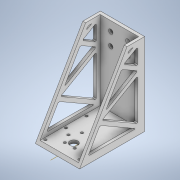
# Autodesk Inventor part: Top
Saved by Autodesk Inventor 2020 (Build 240168000, 168)
## iProperties
Created: 2019-08-01
Part Number: Top
Material: Generic
Document SubType Name: Modeling
Designer: Alex
Density: 1 g/cm^3
Appearance: Default
Author: Alex
Autodesk Inventor part; units mm, degrees
ref_plane "YZ Plane" through (0, 0, 0) normal (1, 0, 0) x (0, 1, 0)
ref_plane "XZ Plane" through (0, 0, 0) normal (0, 1, 0) x (-1, 0, 0)
ref_plane "XY Plane" through (0, 0, 0) normal (0, 0, 1) x (1, 0, 0)
sketch "Sketch1" plane through (0, 0, 0) normal (0, 1, 0) x (-1, 0, 0)
  line L0 (-35, -50) -> (35, -50)
  line L1 (35, -50) -> (35, 50)
  line L2 (35, 50) -> (-35, 50)
  line L3 (-35, 50) -> (-35, -50)
  line L4 (-35, -50) -> (35, 50) construction
  line L5 (35, -50) -> (-35, 50) construction
  point P0 (0, 0)
  dimension "d0" = 70
  dimension "d1" = 100
  constraints: 12 end point, 2 midpoint, 2 parallel, 1 horizontal, 1 perpendicular
  measures "d0" distance of L2.end L1.end
  measures "d1" distance of L1.end L0.end
extrude "Extrusion1" add sketch "Sketch1" along normal blind 5
sketch "Sketch2" plane through (0, 5, 0) normal (0, 1, 0) x (1, 0, 0)
  line L0 (35, -50) -> (35, 50) construction
  line L1 (35, 50) -> (-35, 50) construction
  line L2 (-35, 50) -> (-35, -50) construction
  line L3 (-35, -50) -> (35, -50) construction
  line L4 (-35, -50) -> (35, -50) construction
  line L5 (35, 50) -> (-35, 50) projected
  line L6 (-35, -50) -> (-35, 50)
  line L7 (-35, 50) -> (35, 50)
  line L8 (35, -50) -> (35, 50) projected
  line L9 (35, 50) -> (35, -50)
  line L10 (35, -50) -> (30.5, -50)
  line L11 (30.5, -50) -> (30.5, 45)
  line L12 (30.5, 45) -> (-30.5, 45)
  line L13 (-30.5, 45) -> (-30.5, -50)
  line L14 (-35, -50) -> (-30.5, -50)
  line L15 (0, 70) -> (0, -70) construction
  point P0 (0, 0)
  dimension "d5" = 5
  dimension "d6" = 4.5
  constraints: 16 end point, 4 perpendicular, 2 collinear, 2 point on line, 1 vertical, 1 other
  measures "d5" distance between parallel lines of L1 L12
  measures "d6" distance between parallel lines of L2 L13
extrude "Extrusion2" add sketch "Sketch2" along normal blind 125
draft "FaceDraft1" angle 30 pull direction (0, 1, 0) fixed plane through (10.1667, 5, -13.3333) normal (0, 1, 0) faces at (33.5, 45, 50)
sketch "Sketch3" plane through (0, 5, 0) normal (0, 1, 0) x (1, 0, 0)
  line L0 (-30.5, 45) -> (-30.5, -50) construction
  line L1 (-30.5, -50) -> (30.5, -50) construction
  line L2 (30.5, -50) -> (30.5, 45) construction
  line L3 (30.5, 45) -> (-30.5, 45) construction
  line L4 (-35, -52.8868) -> (35, -52.8868) construction
  line L5 (35, -52.8868) -> (35, 22.1688) construction
  line L6 (30.5, -50) -> (30.5, 22.1688) construction
  line L7 (-30.5, -50) -> (30.5, -50) construction
  line L8 (-30.5, -50) -> (-30.5, 22.1688) construction
  line L9 (-35, -52.8868) -> (-35, 22.1688) construction
  line L10 (30.5, 45) -> (30.5, 22.1688) construction
  line L11 (35, 50) -> (-35, 50) construction
  line L12 (-30.5, 22.1688) -> (-30.5, 45) construction
  line L13 (-30.5, 45) -> (30.5, 45) construction
  circle A0 centre (0, -20) radius 15.5 construction
  line L14 (-35, 50) -> (-35, 22.1688) projected
  line L15 (-35, 22.1688) -> (-30.5, 22.1688) projected
  line L16 (30.5, 22.1688) -> (35, 22.1688) projected
  line L17 (35, 22.1688) -> (35, 50) projected
  line L18 (30.5, 22.1688) -> (35, 22.1688) projected
  line L19 (-35, 22.1688) -> (-30.5, 22.1688) projected
  circle A1 centre (0, -20) radius 19.5 construction
  point P0 (0, 0)
  point P1 (0, 45)
  point P2 (-7.75, -6.5766)
  point P3 (-15.5, -20)
  point P4 (-7.75, -33.4234)
  point P5 (7.75, -33.4234)
  point P6 (15.5, -20)
  point P7 (7.75, -6.5766)
  dimension "d10" = 31
  dimension "d13" = 360
  dimension "d15" = 30
  dimension "d51" = 39
  constraints: 2 coincident, 1 centre point, 1 horizontal alignment, 1 midpoint, 1 vertical alignment, 10 other
  measures "d15" distance from line of L1 point (0, -20)
  measures "d51" diameter of A1
hole "Hole1" at (-7.75, 5, 6.5766) at (-15.5, 5, 20) at (-7.75, 5, 33.4234) at (7.75, 5, 33.4234) at (15.5, 5, 20) at (7.75, 5, 6.5766) direction (0, -1, 0) diameter 4 depth 5
sketch "Sketch4" plane through (35, 0, -50) normal (0, 0, -1) x (-1, 0, 0)
  line L0 (0, 0) -> (70, 0) construction
  line L1 (70, 0) -> (70, 130) construction
  line L2 (0, 130) -> (70, 130) construction
  line L3 (0, 0) -> (0, 130) construction
  line L4 (35, 130) -> (35, 0) construction
  point P0 (21.5, 115)
  point P1 (21.5, 95)
  point P2 (48.5, 115)
  point P3 (48.5, 95)
  dimension "d23" = 27
  dimension "d24" = 15
  dimension "d25" = 20
  constraints: 2 end point, 2 horizontal alignment, 2 vertical alignment, 1 midpoint, 1 perpendicular, 1 symmetric about line
  measures "d23" distance of point (48.5, 115) point (21.5, 115)
  measures "d24" distance from line of L2 point (21.5, 115)
  measures "d25" distance of point (21.5, 115) point (21.5, 95)
hole "Hole2" at (13.5, 115, -50) at (13.5, 95, -50) at (-13.5, 115, -50) at (-13.5, 95, -50) direction (0, 0, 1) diameter 7 end through all
sketch "Sketch5" plane through (0, 5, 0) normal (0, 1, 0) x (1, 0, 0)
  circle A0 centre (15.5, -20) radius 2 construction
  circle A1 centre (-7.75, -33.4234) radius 2 construction
  circle A2 centre (-7.75, -6.5766) radius 2 construction
  circle A3 centre (-15.5, -20) radius 2 construction
  circle A4 centre (7.75, -33.4234) radius 2 construction
  circle A5 centre (7.75, -6.5766) radius 2 construction
  line L0 (30.5, -50) -> (30.5, 45) construction
  line L1 (30.5, 45) -> (-30.5, 45) construction
  line L2 (-30.5, 45) -> (-30.5, -50) construction
  line L3 (-30.5, -50) -> (30.5, -50) construction
  circle A6 centre (0, -20) radius 15.5 construction
  circle A7 centre (0, -20) radius 19.5 construction
  circle A8 centre (0, -27) radius 6.25
  line L4 (-30.5, -50) -> (30.5, -50) construction
  point P0 (0, 0)
  point P1 (0, -39.5)
  point P2 (0, -33.25)
  point P3 (0, -50)
  dimension "d33" = 39
  dimension "d34" = 12.5
  dimension "d62" = 6.25
  constraints: 5 vertical alignment, 1 coincident, 1 midpoint, 4 other
  measures "d62" distance of point (0, -33.25) point (0, -39.5)
extrude "Extrusion3" cut sketch "Sketch5" against normal blind 5
sketch "Sketch6" plane through (-35, 0, -50) normal (-1, 0, 0) x (0, 0, 1)
  line L0 (0, 0) -> (102.8868, 0) construction
  line L1 (102.8868, 0) -> (27.8312, 130) construction
  line L2 (0, 130) -> (27.8312, 130) construction
  line L3 (0, 0) -> (0, 130) construction
  line L4 (5, 5) -> (100, 5) construction
  line L5 (5, 5) -> (5, 130) construction
  line L6 (27.8312, 130) -> (5, 130) construction
  line L7 (100, 5) -> (27.8312, 130) construction
  line L8 (0, 0) -> (0, 130) projected
  line L9 (11, 124) -> (11, 11) construction
  line L10 (11, 11) -> (89.6077, 11) construction
  line L11 (89.6077, 11) -> (24.3671, 124) construction
  line L12 (24.3671, 124) -> (11, 124) construction
  line L13 (14, 11) -> (70.7058, 43.7391) construction
  line L14 (14, 11) -> (79.4782, 11) construction
  line L15 (11, 16.1962) -> (67.7058, 48.9352) construction
  line L16 (67.7058, 48.9352) -> (11, 81.6743) construction
  line L17 (11, 88.6025) -> (61.7058, 59.3275) construction
  line L18 (11, 88.6025) -> (36.3529, 103.24) construction
  line L19 (11, 95.5307) -> (33.3529, 108.4362) construction
  line L20 (33.3529, 108.4362) -> (11, 121.3416) construction
  line L21 (11, 128.2698) -> (27.3529, 118.8285) construction
  line L22 (11, 16.1962) -> (14, 11) construction
  line L23 (16, 11) -> (87.6077, 11)
  line L24 (71.7058, 42.007) -> (88.6077, 12.7321)
  line L25 (68.9737, 42.7391) -> (15.7321, 12)
  line L26 (12.7321, 17.1962) -> (65.9737, 47.9352)
  line L27 (12.7321, 80.6743) -> (65.9737, 49.9352)
  line L28 (11, 79.6743) -> (11, 18.1962)
  line L29 (12.7321, 89.6025) -> (34.6208, 102.24)
  line L30 (60.7058, 61.0596) -> (37.3529, 101.508)
  line L31 (12.7321, 87.6025) -> (59.9737, 60.3275)
  line L32 (12.7321, 96.5307) -> (31.6208, 107.4362)
  line L33 (25.3671, 122.2679) -> (26.3529, 120.5605)
  line L34 (31.6208, 109.4362) -> (12.7321, 120.3416)
  line L35 (11, 119.3416) -> (11, 97.5307)
  line L36 (11, 128.2698) -> (11, 122)
  line L37 (13, 124) -> (22.3671, 124)
  line L38 (11, 128.2698) -> (25.6208, 119.8285)
  line L39 (22.3671, 124) -> (25.3671, 122.2679)
  line L40 (25.6208, 119.8285) -> (26.3529, 120.5605)
  line L41 (13, 124) -> (11, 122)
  line L42 (12.7321, 120.3416) -> (11, 119.3416)
  line L43 (31.6208, 107.4362) -> (31.6208, 109.4362)
  line L44 (11, 97.5307) -> (12.7321, 96.5307)
  line L45 (34.6208, 102.24) -> (37.3529, 101.508)
  line L46 (34.6208, 102.24) -> (37.3529, 101.508)
  line L47 (12.7321, 87.6025) -> (12.7321, 89.6025)
  line L48 (59.9737, 60.3275) -> (60.7058, 61.0596)
  line L49 (12.7321, 17.1962) -> (11, 18.1962)
  line L50 (65.9737, 49.9352) -> (65.9737, 47.9352)
  line L51 (11, 79.6743) -> (12.7321, 80.6743)
  line L52 (88.6077, 12.7321) -> (87.6077, 11)
  line L53 (68.9737, 42.7391) -> (71.7058, 42.007)
  line L54 (15.7321, 12) -> (16, 11)
  point P0 (18.3956, 124)
  dimension "d64" = 6
  dimension "d65" = 30
  dimension "d66" = 6
  dimension "d67" = 6
  dimension "d68" = 6
  dimension "d69" = 6
  dimension "d71" = 60
  dimension "d72" = 60
  dimension "d75" = 2
  dimension "d76" = 2
  dimension "d77" = 2
  dimension "d78" = 2
  dimension "d79" = 2
  dimension "d80" = 2
  dimension "d81" = 2
  dimension "d82" = 2
  dimension "d83" = 2
  dimension "d84" = 2
  dimension "d85" = 2
  dimension "d86" = 2
  dimension "d87" = 2
  dimension "d88" = 2
  dimension "d89" = 2
  dimension "d90" = 2
  dimension "d91" = 2
  dimension "d92" = 2
  dimension "d93" = 2
  dimension "d94" = 2
  dimension "d95" = 2
  dimension "d96" = 2
  dimension "d97" = 2
  dimension "d98" = 2
  dimension "d99" = 2
  dimension "d100" = 2
  dimension "d101" = 2
  dimension "d102" = 2
  dimension "d103" = 2
  dimension "d104" = 2
  dimension "d105" = 2
  dimension "d106" = 2
  constraints: 92 end point, 47 point on line, 6 collinear, 6 perpendicular, 5 parallel, 1 equal length, 1 horizontal, 3 other
  measures "d64" distance between parallel lines of L5 L9
  measures "d65" angle of L14 L13
  measures "d66" distance between parallel lines of L15 L13
  measures "d67" distance between parallel lines of L17 L16
  measures "d68" distance between parallel lines of L18 L19
  measures "d69" distance between parallel lines of L21 L20
  measures "d71" angle of L15 L16
  measures "d72" angle of L19 L20
  measures "d75" distance of L37.end L11.end
  measures "d76" distance of L33.start L11.end
  measures "d77" distance of L38.end L21.end
  measures "d78" distance of L33.end L21.end
  measures "d79" distance of L37.start L9.start
  measures "d80" distance of L36.end L9.start
  measures "d81" distance of L34.end L20.end
  measures "d82" distance of L35.start L20.end
  measures "d83" distance of L32.end L19.end
  measures "d84" distance of L34.start L19.end
  measures "d85" distance of L35.end L19.start
  measures "d86" distance of L32.start L19.start
  measures "d87" distance of L45.start L18.end
  measures "d88" distance of L45.end L18.end
  measures "d89" distance of L29.end point (36.353, 103.24)
  measures "d90" distance of L30.end point (36.353, 103.24)
  measures "d91" distance of L31.start L17.start
  measures "d92" distance of L29.start L17.start
  measures "d93" distance of L31.end L17.end
  measures "d94" distance of L30.start L17.end
  measures "d95" distance of L26.start L15.start
  measures "d96" distance of L28.end L15.start
  measures "d97" distance of L27.end L15.end
  measures "d98" distance of L26.end L15.end
  measures "d99" distance of L28.start L16.end
  measures "d100" distance of L27.start L16.end
  measures "d101" distance of L24.end L10.end
  measures "d102" distance of L23.end L10.end
  measures "d103" distance of L25.start L13.end
  measures "d104" distance of L24.start L13.end
  measures "d105" distance of L25.end L13.start
  measures "d106" distance of L23.start L13.start
sketch "Sketch7" plane through (0, 5, 0) normal (0, 1, 0) x (1, 0, 0)
  circle A0 centre (0, -20) radius 19.5 construction
  circle A1 centre (0, -20) radius 15.5 construction
  line L0 (0, 70) -> (0, -70) construction
  line L1 (-30.5, -50) -> (30.5, -50) construction
  line L2 (-30.5, 45) -> (30.5, 45) projected
  line L3 (-27, -45) -> (-27, -12.5) construction
  line L4 (-27, -12.5) -> (-27, 20) construction
  point P0 (0, 0)
  point P1 (27, -12.5)
  point P2 (27, -45)
  point P3 (27, 20)
  dimension "d52" = 54
  dimension "d54" = 5
  dimension "d63" = 25
  constraints: 4 end point, 4 vertical alignment, 3 horizontal alignment, 2 vertical, 1 collinear, 1 symmetric about line
  measures "d52" distance of point (27, -12.5) L3.end
  measures "d54" distance from line of L1 L3.start
  measures "d63" distance from line of L4.end L2
hole "Hole3" at (-27, 5, 12.5) at (27, 5, 12.5) at (-27, 5, 45) at (27, 5, 45) at (27, 5, -20) at (-27, 5, -20) direction (0, -1, 0) diameter 4 depth 5
extrude "Extrusion5" cut sketch "Sketch6" against normal through all contours L54 L25 L53 L24 L52 L23 | L49 L28 L51 L27 L50 L26 | L29 L45 L30 L48 L31 L47 | L44 L35 L42 L34 L43 L32 | L33 L40 L38 L37 L39
equation "\"d66\" = d64"
equation "\"d67\" = d64"
equation "\"d68\" = d64"
equation "\"d69\" = d64"
equation "\"d71\" = 2 * d65"
equation "\"d72\" = 2 * d65"
equation "\"d76\" = d75"
equation "\"d78\" = d77"
equation "\"d80\" = d79"
equation "\"d82\" = d81"
equation "\"d84\" = d83"
equation "\"d86\" = d85"
equation "\"d88\" = d87"
equation "\"d90\" = d89"
equation "\"d92\" = d91"
equation "\"d93\" = d91"
equation "\"d94\" = d93"
equation "\"d95\" = d91"
equation "\"d96\" = d95"
equation "\"d98\" = d97"
equation "\"d100\" = d99"
equation "\"d102\" = d101"
equation "\"d103\" = d101"
equation "\"d104\" = d103"
equation "\"d105\" = d101"
equation "\"d106\" = d105"
body "Solid1"
